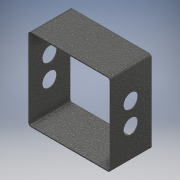
# Autodesk Inventor part: Stackbox-110mm
Saved by Autodesk Inventor 2017 (Build 210142000, 142)
## iProperties
Created: 2017-10-10
Part Number: Stackbox-110mm
Material: Generic
Document SubType Name: Modeling
Designer: Kathryn Rosie
Density: 1 g/cm^3
Appearance: Black
Author: Kathryn Rosie
Autodesk Inventor part; units mm, degrees
ref_plane "YZ Plane" through (0, 0, 0) normal (1, 0, 0) x (0, 1, 0)
ref_plane "XZ Plane" through (0, 0, 0) normal (0, 1, 0) x (-1, 0, 0)
ref_plane "XY Plane" through (0, 0, 0) normal (0, 0, 1) x (1, 0, 0)
sketch "Sketch1" plane through (0, 0, 0) normal (0, 1, 0) x (-1, 0, 0)
  line L0 (-280, 300) -> (280, 300)
  line L1 (300, 280) -> (300, -280)
  line L2 (280, -300) -> (-280, -300)
  line L3 (-300, -280) -> (-300, 280)
  line L4 (-300, 300) -> (300, -300) construction
  line L5 (300, 300) -> (-300, -300) construction
  arc A0 (300, 280) -> (280, 300) centre (280, 280) ccw
  arc A1 (280, -300) -> (300, -280) centre (280, -280) ccw
  arc A2 (-300, -280) -> (-280, -300) centre (-280, -280) ccw
  arc A3 (-280, 300) -> (-300, 280) centre (-280, 280) ccw
  line L6 (280, 294) -> (-280, 294)
  arc A4 (-280, 294) -> (-294, 280) centre (-280, 280) ccw
  line L7 (-294, 280) -> (-294, -280)
  arc A5 (-294, -280) -> (-280, -294) centre (-280, -280) ccw
  line L8 (-280, -294) -> (280, -294)
  arc A6 (280, -294) -> (294, -280) centre (280, -280) ccw
  line L9 (294, -280) -> (294, 280)
  arc A7 (294, 280) -> (280, 294) centre (280, 280) ccw
  point P0 (0, 0)
  dimension "d0" = 600
  dimension "d1" = 600
  dimension "d2" = 20
  dimension "d3" = 6
  constraints: 20 end point, 16 point on circle, 8 centre point, 8 point on line, 8 tangent, 4 parallel, 3 equal radius, 2 midpoint, 2 perpendicular, 1 horizontal, 7 other
  measures "d0" distance of L4.end L5.end
  measures "d1" distance of L5.start L4.end
  measures "d2" radius of A0
  measures "d3" distance between parallel lines of L0 L6
extrude "Extrusion1" add sketch "Sketch1" along normal blind 300
sketch "Sketch2" plane through (300, 0, 280) normal (1, 0, 0) x (0, 0, -1)
  line L0 (0, 0) -> (0, 300) projected
  line L1 (0, 150) -> (560, 150) construction
  line L2 (560, 0) -> (560, 300) projected
  point P0 (280, 0)
  point P1 (200, 150)
  point P2 (360, 150)
  dimension "d8" = 160
  dimension "d28" = 200
  constraints: 2 end point, 2 midpoint, 2 point on line
  measures "d8" distance of point (360, 150) point (200, 150)
  measures "d28" distance from line of L0 point (200, 150)
hole "Hole1" at (300, 150, 80) at (300, 150, -80) direction (-1, 0, 0) diameter 110 end through all
body "Solid1"
